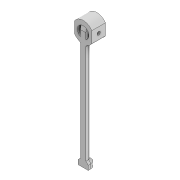
# Autodesk Inventor part: endoscope_holder_2
Saved by Autodesk Inventor 2022 (Build 260153000, 153)
## iProperties
Created: 2021-07-04
Part Number: endoscope_holder_2
Material: Generic
Document SubType Name: Modeling
Designer: dsdan
Density: 1 g/cm^3
Appearance: Default
Author: dsdan
Autodesk Inventor part; units mm, degrees
ref_plane "YZ Plane" through (0, 0, 0) normal (1, 0, 0) x (0, 1, 0)
ref_plane "XY Plane" through (0, 0, 0) normal (0, 0, 1) x (1, 0, 0)
sketch "Sketch1" plane through (0, 0, 0) normal (0, 1, 0) x (-1, 0, 0)
  arc A0 (-3, 0) -> (3, 0) centre (0, 0) ccw
  line L0 (-3, 0) -> (3, 0) construction
  line L1 (3, 0) -> (3, 3)
  line L2 (3, 3) -> (-3, 3)
  line L3 (-3, 3) -> (-3, 0)
  dimension "d0" = 6
  constraints: 8 end point, 3 tangent, 2 parallel, 2 point on circle, 1 centre point, 1 coincident, 1 horizontal, 1 perpendicular
  measures "d0" diameter of A0
extrude "Extrusion1" add sketch "Sketch1" against normal blind 250
sketch "Sketch10" plane through (3, -250, 3) normal (1, 0, 0) x (0, 0, -1)
  line L0 (0, 250) -> (0, 0) projected
  line L1 (0, 0) -> (6, 1.058)
  line L2 (6, 250) -> (6, 0) projected
  line L3 (3, 0) -> (6, 0) projected
  line L4 (3, 0) -> (0, 0) projected
  point P0 (3, 250)
  dimension "d56" = 10
  constraints: 2 end point, 1 point on line
  measures "d56" angle of L3 L1
extrude "Extrusion10" cut sketch "Sketch10" along normal through all both and the other way through all
sketch "Sketch11" plane through (-3, -250, 3) normal (0, -0.9848078, -0.1736482) x (1, 0, 0)
  line L0 (6, 0) -> (6, -3.0463) projected
  line L1 (6, 0) -> (0, 0) projected
  line L2 (0, -3.0463) -> (0, 0) projected
  ellipse E0 centre (3, -3.0463) end of major axis (3, 0) minor radius 3 (0, -3.0463) -> (6, -3.0463) ccw projected
  point P0 (3, -46.3665)
  constraints: 1 other
extrude "Extrusion11" add sketch "Sketch11" along normal blind 10
sketch "Sketch2" plane through (0, 0, 0) normal (1, 0, 0) x (0, 1, 0)
  line L0 (-259.0546, -3.2365) -> (-261.0242, -3.5838)
  line L1 (-261.0242, -3.5838) -> (-261.6407, -0.0877)
  line L2 (-260.0184, 2.2292) -> (-259.0546, -3.2365)
  line L3 (-260.0184, 2.2292) -> (-278.7297, -1.0701)
  line L4 (-278.7297, -1.0701) -> (-278.3824, -3.0397)
  line L5 (-278.3824, -3.0397) -> (-261.6407, -0.0877)
  line L6 (-259.3191, -1.7365) -> (-258.7901, -4.7365) projected
  line L7 (-259.0546, -3.2365) -> (-236.7514, 0.6962) construction
  point P0 (0, 0)
  dimension "d5" = 17
  dimension "d6" = 2
  dimension "d38" = 2
  dimension "d61" = 7.1
  constraints: 14 end point, 3 perpendicular, 2 parallel, 1 collinear, 1 midpoint
  measures "d5" distance between parallel lines of L1 L4
  measures "d6" distance between parallel lines of L2 L1
  measures "d38" distance between parallel lines of L5 L3
  measures "d61" diameter of L5 L7
revolve "Revolution1" add sketch "Sketch2" angle 280 mid plane about axis through (0, -259.0546, -3.2365) along (0, 0.9848078, 0.1736482)
sketch "Sketch3" plane through (0, -259.6366, 0.0641) normal (0, -0.9848078, -0.1736482) x (1, 0, 0)
  circle A0 centre (0, -1.8283) radius 1.2
  ellipse E0 centre (0, -1.8283) end of major axis (0, 1.2179) minor radius 3 (-3, -1.8283) -> (-1.1, -4.6624) ccw projected
  line L0 (1.2, -1.8283) -> (1.2, -12.8275)
  line L1 (1.2, -12.8275) -> (-1.2, -12.8275)
  line L2 (-1.2, -12.8275) -> (-1.2, -1.8283)
  dimension "d62" = 2.4
  constraints: 6 end point, 2 perpendicular, 2 point on circle, 2 tangent, 1 centre point, 1 vertical, 2 other
  measures "d62" diameter of A0
extrude "Extrusion7" cut sketch "Sketch3" along normal mid plane 21
sketch "Sketch12" plane through (0, 0, 0) normal (0, 1, 0) x (1, 0, 0)
  arc A0 (-1.2, 2.7495) -> (-3, 0) centre (0, 0) ccw projected
  circle A1 centre (0, 0) radius 1.2
  line L0 (1.2, 0) -> (1.2, 5.3669)
  line L1 (1.2, 5.3669) -> (-1.2, 5.3669)
  line L2 (-1.2, 5.3669) -> (-1.2, 0)
  dimension "d63" = 2.4
  constraints: 6 end point, 2 perpendicular, 2 point on circle, 2 tangent, 1 centre point, 1 coincident, 1 vertical
  measures "d63" diameter of A1
extrude "Extrusion12" cut sketch "Sketch12" against normal blind 235
ref_plane "Work Plane3" through (0, 0, 0) normal (0, 0, 1) x (1, 0, 0)
sketch "Sketch8" plane through (0, 0, 3) normal (0, 0, 1) x (1, 0, 0)
  circle A0 centre (0, 9) radius 6.35
  circle A1 centre (0, 9) radius 11.35
  line L0 (-9.5, 2.7893) -> (-9.5, 15.2107)
  line L1 (9.5, 2.7893) -> (9.5, 15.2107)
  point P0 (0, 0)
  dimension "d44" = 12.7
  dimension "d45" = 5
  dimension "d46" = 19
  constraints: 4 end point, 4 point on circle, 2 centre point, 2 horizontal alignment, 1 coincident, 1 parallel, 1 vertical alignment
  measures "d44" diameter of A0
  measures "d45" radial gap between concentric circles of A1 A0
  measures "d46" distance between parallel lines of L0 L1
extrude "Extrusion8" add sketch "Sketch8" against normal blind 15 contours L1 A1 L0
chamfer "Chamfer3" distance 0.4 angle 45 2 edges at (0, -278.7297, -1.0701) (0, -278.3824, -3.0397)
fillet "Fillet2" radius 2 2 edges at (2.5693, -2.0554, -1.5487) (-2.5686, -2.0555, -1.5499)
chamfer "Chamfer6" distance 2.3 angle 45 3 edges at (0, -261.4971, -0.902) (1.2, -261.0323, -3.538) (-1.2, -261.0323, -3.538)
sketch "Sketch9" plane through (9.5, 15.2107, -12) normal (1, 0, 0) x (0, -1, 0)
  circle A0 centre (6.2107, -7.5) radius 1.8
  line L0 (12.4214, -15) -> (12.4214, 0) projected
  line L1 (0, 0) -> (12.4214, 0) projected
  point P0 (15.2107, -12)
  point P1 (12.4214, -7.5)
  point P2 (12.4214, 15)
  point P3 (6.2107, 0)
  dimension "d53" = 3.6
  constraints: 2 midpoint, 1 centre point, 1 horizontal alignment, 1 vertical alignment
  measures "d53" diameter of A0
extrude "Extrusion9" cut sketch "Sketch9" against normal up to surface round surface about axis through (0, 9, 3) along (0, 0, -1) radius 6.35 far side no
chamfer "Chamfer7" distance 3 angle 45 4 edges at (-3, -259.5836, -0.2365) (-2.5981, -259.0546, -3.2365) (2.5981, -259.0546, -3.2365) (3, -259.5836, -0.2365)
chamfer "Chamfer8" distance 0.5 angle 45 1 edges at (0, -259.8481, 1.2635)
ref_plane "Work Plane5" through (0, -115, 0) normal (0, 1, 0) x (-1, 0, 0)
ref_plane "Work Plane4" through (0, -120, 0) normal (0, 1, 0) x (-1, 0, 0)
sketch "Sketch13" plane through (0, -115, 0) normal (0, 1, 0) x (-1, 0, 0)
  line L0 (1.2, -2.7495) -> (1.2, 0) projected
  arc A0 (1.2, 0) -> (-1.2, 0) centre (0, 0) ccw projected
  line L1 (-1.2, 0) -> (-1.2, -2.7495) projected
  arc A1 (-3, 0) -> (-1.2, -2.7495) centre (0, 0) ccw projected
  line L2 (-3, 0) -> (-3, 3) projected
  line L3 (-3, 3) -> (3, 3) projected
  line L4 (3, 3) -> (3, 0) projected
  arc A2 (1.2, -2.7495) -> (3, 0) centre (0, 0) ccw projected
  line L5 (5.5, 5.5) -> (-5.5, 5.5)
  line L6 (-5.5, 5.5) -> (-5.5, 0)
  arc A3 (-5.5, 0) -> (-1.65, -5.2467) centre (0, 0) ccw
  arc A4 (-1.65, -5.2467) -> (5.5, 0) centre (0, 0) ccw
  line L7 (5.5, 0) -> (5.5, 5.5)
  line L8 (3, 3) -> (3, 1.7845) projected
  line L9 (3, 3) -> (5.5, 3)
  line L10 (-3, 3) -> (-3, 1.7845) projected
  line L11 (-3, 3) -> (-5.5, 3)
  line L12 (-1.2, -2.7495) -> (-2.4543, -4.922)
  line L13 (1.2, -2.7495) -> (1.2, -3.9651) projected
  line L14 (1.2, -2.7495) -> (2.4543, -4.922)
  dimension "d77" = 2.5
  dimension "d78" = 30
  dimension "d79" = 30
  constraints: 14 end point, 6 point on circle, 3 point on line, 2 centre point, 1 perpendicular, 4 other
  measures "d77" distance between parallel lines of L3 L5
  measures "d78" angle of L13 L14
  measures "d79" angle of L13 L12
extrude "Extrusion13" add sketch "Sketch13" against normal up to surface (5 mm away) contours A2 L4 L9 L7 A4 L14 | L12 A3 L6 L11 L2 A1
chamfer "Chamfer9" distance 2.5 angle 45 4 edges at (3, -115, 1.5) (2.51, -115, -1.6432) (-3, -115, 1.5) (-2.51, -115, -1.6432)
mirror "Mirror1" about plane through (0, -120, 0) normal (0, 1, 0) of "Chamfer9", "Extrusion13", "Extrusion11", "Fillet2", "Extrusion12", "Extrusion1", "Extrusion8"
split body "Split1" result two bodies by plane through (0, -120, 0) normal (0, 1, 0) first body at (1, -39.7522, 2.5)
body "Solid2"
body "Solid3"
